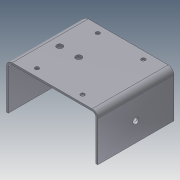
# Autodesk Inventor part: GE-12025
Saved by Autodesk Inventor 2012 (Build 160160000, 160)
## iProperties
Created: 2011-06-06
Part Number: GE-12025
Document SubType Name: Modeling
Designer: dfoster
Density: 7.85 g/cm^3
Material: Steel
Mass: 872.396 g
Surface Area: 764.225 cm^2
Volume: 111.133 cm^3
Description: Bridge Holder
Title: Bridge Holder
Author: dfoster
Autodesk Inventor part; units mm, degrees
ref_plane "YZ Plane" through (0, 0, 0) normal (1, 0, 0) x (0, 1, 0)
ref_plane "XZ Plane" through (0, 0, 0) normal (0, 1, 0) x (-1, 0, 0)
ref_plane "XY Plane" through (0, 0, 0) normal (0, 0, 1) x (1, 0, 0)
sketch "Sketch1" plane through (0, 0, 0) normal (0, 0, 1) x (1, 0, 0)
  line L0 (0, 0) -> (0, 66.675)
  line L1 (9.525, 76.2) -> (142.875, 76.2)
  line L2 (152.4, 66.675) -> (152.4, 0)
  line L3 (152.4, 0) -> (149.3622, 0)
  line L4 (149.3622, 0) -> (149.3622, 66.8122)
  line L5 (143.0122, 73.1622) -> (9.3878, 73.1622)
  line L6 (3.0378, 66.8122) -> (3.0378, 0)
  line L7 (3.0378, 0) -> (0, 0)
  arc A0 (9.3878, 73.1622) -> (3.0378, 66.8122) centre (9.3878, 66.8122) ccw
  arc A1 (149.3622, 66.8122) -> (143.0122, 73.1622) centre (143.0122, 66.8122) ccw
  arc A2 (9.525, 76.2) -> (0, 66.675) centre (9.525, 66.675) ccw
  arc A3 (152.4, 66.675) -> (142.875, 76.2) centre (142.875, 66.675) ccw
  point P0 (0, 76.2)
  point P1 (152.4, 76.2)
  dimension "d0" = 76.2
  dimension "d1" = 3.0378
  dimension "d2" = 3.0378
  dimension "d3" = 152.4
  dimension "d4" = 6.35
  dimension "d5" = 9.525
  constraints: 16 end point, 8 point on circle, 8 tangent, 6 parallel, 4 centre point, 4 point on line, 2 equal length, 2 equal radius, 1 perpendicular, 1 vertical
  measures "d0" distance of L0.start point (0, 76.2)
  measures "d1" distance between parallel lines of L6 L0
  measures "d2" distance between parallel lines of L5 L1
  measures "d3" distance of point (0, 76.2) point (152.4, 76.2)
  measures "d4" radius of A0
  measures "d5" radius of A2
extrude "Extrusion1" add sketch "Sketch1" along normal blind 127
hole "Hole1" at (25.4, 76.2, 63.5) direction (0, -1, 0) diameter 9.906 end through all
pattern_linear "Rectangular Pattern1" count 2 spacing 31.75 along (1, 0, 0) of "Hole1"
hole "Hole2" at (0, 31.75, 63.5) direction (1, 0, 0) diameter 9.906 end through all
hole "Hole3" at (38.1, 73.1622, 12.7) direction (0, 1, 0) diameter 6.731 depth 25.4 tip angle 118
pattern_linear "Rectangular Pattern2" count 2 spacing 76.2 along (1, 0, 0) count 2 spacing 101.6 along (0, 0, 1) of "Hole3"
equation "\"d2\" = d1"
body "Solid1"
